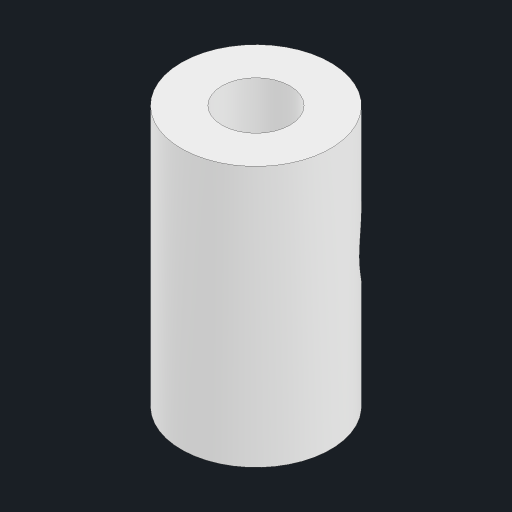
# Autodesk Inventor part: motor_shaft_adapter
Saved by Autodesk Inventor 2023 (Build 270158000, 158)
## iProperties
Created: 2024-04-12
Part Number: motor_shaft_adapter
Material: ABS Plastic
Document SubType Name: Modeling
Designer: szymo
Density: 1.06 g/cm^3
Appearance: Smooth - White
Author: szymo
Autodesk Inventor part; units mm, degrees
ref_plane "YZ Plane" through (0, 0, 0) normal (1, 0, 0) x (0, 1, 0)
ref_plane "XZ Plane" through (0, 0, 0) normal (0, 1, 0) x (-1, 0, 0)
sketch "Sketch1" plane through (0, 0, 0) normal (0, 1, 0) x (-1, 0, 0)
  circle A0 centre (-2.575, 2.575) radius 1.175
  circle A1 centre (-2.575, 2.575) radius 2.575
  line L0 (0, 0) -> (-7.3028, 0) construction
  line L1 (0, 0) -> (0, 4.3038) construction
  dimension "d0" = 2.35
  dimension "d1" = 5.15
  constraints: 4 end point, 2 centre point, 2 coincident, 2 horizontal, 2 tangent, 2 vertical
  measures "d0" diameter of A0
  measures "d1" diameter of A1
extrude "Extrusion1" add sketch "Sketch1" along normal blind 9
ref_plane "Work Plane1" through (2.575, 0, 1.4) normal (0, 0, 1) x (1, 0, 0)
ref_plane "screwMaxDist" through (2.575, 0, 1.9) normal (0, 0, 1) x (1, 0, 0)
sketch "Sketch2" plane through (0, 0, 0) normal (0, 0, 1) x (1, 0, 0)
  line L0 (5.15, 9) -> (0, 9) projected
  circle A0 centre (2.575, 4.85) radius 2.15
  line L1 (5.15, 9) -> (0, 9) projected
  line L2 (5.15, 0) -> (0, 0) projected
  line L3 (0, 0) -> (0, 9) projected
  line L4 (0, 7) -> (5.15, 7)
  line L5 (5.15, 0) -> (5.15, 9) projected
  dimension "d5" = 4.3
  dimension "d15" = 2
  dimension "d16" = 2.575
  dimension "d17" = 2.575
  constraints: 2 end point, 2 point on line, 1 centre point, 1 parallel, 1 tangent
  measures "d5" diameter of A0
  measures "d15" distance between parallel lines of L0 L4
  measures "d16" distance from line of A0.centre L5
  measures "d17" distance from line of L3 A0.centre
extrude "Extrusion2" cut sketch "Sketch2" along normal up to surface (1.9 mm away) contours A0
equation "\"d16\" = d17"
body "Solid1"
